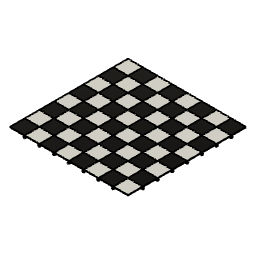
Skak v6 (Autodesk Fusion 360 design; units mm, degrees)
Autodesk Fusion 360 part; units mm, degrees
sketch "Sketch1" plane through (0, 0, 0) normal (1, 0, 0) x (0, 1, 0) in component "Stifner_X"
  line L0 (2, 4) -> (-2, 4)
  line L1 (-2, 4) -> (-2, 0)
  line L2 (-2, 0) -> (2, 0)
  line L3 (2, 0) -> (2, 4)
  dimension "d190" = 4
  dimension "d191" = 4
  constraint horizontal L0
  constraint vertical L1
  constraint horizontal L2
  constraint vertical L3
  constraint midpoint origin L2
  measures "d190" distance of L0 L2
  measures "d191" distance of L0.start L0.end
extrude "Extrude1" add sketch "Sketch1" along normal blind 324 makes body 1 in component "Stifner_X"
sketch "Sketch5" plane through (0, -2, 0) normal (0, -1, 0) x (1, 0, 0) in component "Stifner_X"
  line L0 (0, 4) -> (0, 0)
  line L1 (0, 0) -> (324, 0)
  line L2 (324, 0) -> (324, 4)
  line L3 (324, 4) -> (0, 4)
  line L4 (40, 4) -> (44, 4)
  line L5 (44, 4) -> (44, 2)
  line L6 (44, 2) -> (40, 2)
  line L7 (40, 2) -> (40, 4)
  line L8 (44, 4) -> (44, 2)
  line L9 (44, 2) -> (40, 2)
  line L10 (40, 2) -> (40, 4)
  line L11 (40, 4) -> (44, 4)
  line L12 (80, 2) -> (80, 4)
  line L13 (84, 2) -> (80, 2)
  line L14 (84, 4) -> (84, 2)
  line L15 (80, 4) -> (84, 4)
  line L16 (120, 2) -> (120, 4)
  line L17 (124, 2) -> (120, 2)
  line L18 (124, 4) -> (124, 2)
  line L19 (120, 4) -> (124, 4)
  line L20 (160, 2) -> (160, 4)
  line L21 (164, 2) -> (160, 2)
  line L22 (164, 4) -> (164, 2)
  line L23 (160, 4) -> (164, 4)
  line L24 (200, 2) -> (200, 4)
  line L25 (204, 2) -> (200, 2)
  line L26 (204, 4) -> (204, 2)
  line L27 (200, 4) -> (204, 4)
  line L28 (240, 2) -> (240, 4)
  line L29 (244, 2) -> (240, 2)
  line L30 (244, 4) -> (244, 2)
  line L31 (240, 4) -> (244, 4)
  line L32 (280, 2) -> (280, 4)
  line L33 (284, 2) -> (280, 2)
  line L34 (284, 4) -> (284, 2)
  line L35 (280, 4) -> (284, 4)
  dimension "d200" = 4
  dimension "d201" = 2
  dimension "d202" = 40
  dimension "d205" = 40
  dimension "d206" = 0
  constraint horizontal L4
  constraint vertical L5
  constraint horizontal L6
  constraint vertical L7
  constraint coincident L3 L4.start
  measures "d200" distance of L4.start L4.end
  measures "d201" distance of L4.start L6.end
  measures "d202" distance of L0 L7
extrude "Extrude2" cut sketch "Sketch5" against normal through all contours L3 L4 L5 L6 L7 L8 L9 L10 L11 | L3 L12 L13 L14 L15 | L3 L32 L33 L34 L35 | L3 L16 L17 L18 L19 | L3 L28 L29 L30 L31 | L3 L20 L21 L22 L23 | L3 L24 L25 L26 L27 bodies 1 in component "Stifner_X"
sketch "Sketch1 (2)" plane through (0, 0, 0) normal (0, 1, 0) x (1, 0, 0) in component "Stifner_Y"
  line L0 (-2, -4) -> (2, -4)
  line L1 (2, -4) -> (2, 0)
  line L2 (2, 0) -> (-2, 0)
  line L3 (-2, 0) -> (-2, -4)
  dimension "d207" = 4
  dimension "d208" = 4
  constraint horizontal L0
  constraint vertical L1
  constraint horizontal L2
  constraint vertical L3
  constraint midpoint origin L2
  measures "d207" distance of L0.start L0.end
  measures "d208" distance of L0.start L2.end
extrude "Extrude1'" add sketch "Sketch1 (2)" along normal blind 324 separate body makes body 2 in component "Stifner_Y"
sketch "Sketch3" plane through (2, 0, 0) normal (1, 0, 0) x (0, 1, 0) in component "Stifner_Y"
  line L0 (0, 4) -> (0, 0)
  line L1 (0, 0) -> (324, 0)
  line L2 (324, 0) -> (324, 4)
  line L3 (324, 4) -> (0, 4)
  line L4 (40, 0) -> (44, 0)
  line L5 (44, 0) -> (44, 2)
  line L6 (44, 2) -> (40, 2)
  line L7 (40, 2) -> (40, 0)
  line L8 (40, 0) -> (44, 0)
  line L9 (44, 0) -> (44, 2)
  line L10 (44, 2) -> (40, 2)
  line L11 (40, 2) -> (40, 0)
  line L12 (84, 2) -> (80, 2)
  line L13 (80, 2) -> (80, 0)
  line L14 (80, 0) -> (84, 0)
  line L15 (84, 0) -> (84, 2)
  line L16 (124, 2) -> (120, 2)
  line L17 (120, 2) -> (120, 0)
  line L18 (120, 0) -> (124, 0)
  line L19 (124, 0) -> (124, 2)
  line L20 (164, 2) -> (160, 2)
  line L21 (160, 2) -> (160, 0)
  line L22 (160, 0) -> (164, 0)
  line L23 (164, 0) -> (164, 2)
  line L24 (204, 2) -> (200, 2)
  line L25 (200, 2) -> (200, 0)
  line L26 (200, 0) -> (204, 0)
  line L27 (204, 0) -> (204, 2)
  line L28 (244, 2) -> (240, 2)
  line L29 (240, 2) -> (240, 0)
  line L30 (240, 0) -> (244, 0)
  line L31 (244, 0) -> (244, 2)
  line L32 (284, 2) -> (280, 2)
  line L33 (280, 2) -> (280, 0)
  line L34 (280, 0) -> (284, 0)
  line L35 (284, 0) -> (284, 2)
  point P0 (84, 2)
  point P1 (80, 2)
  point P2 (124, 2)
  point P3 (120, 2)
  point P4 (164, 2)
  point P5 (160, 2)
  point P6 (204, 2)
  point P7 (200, 2)
  point P8 (244, 2)
  point P9 (240, 2)
  point P10 (284, 2)
  point P11 (280, 2)
  dimension "d209" = 2
  dimension "d210" = 4
  dimension "d211" = 40
  dimension "d214" = 40
  dimension "d215" = 0
  dimension "d233" = 0
  constraint horizontal L4
  constraint vertical L5
  constraint horizontal L6
  constraint vertical L7
  constraint coincident L1 L4.start
  measures "d209" distance of L4.start L6.end
  measures "d210" distance of L4.start L4.end
  measures "d211" distance of L0 L7
  measures "d233" distance of L4
extrude "Extrude2'" cut sketch "Sketch3" against normal through all contours L1 L4 L5 L6 L7 L8 L9 L10 L11 | L1 L32 L33 L34 L35 | L1 L12 L13 L14 L15 | L1 L28 L29 L30 L31 | L1 L16 L17 L18 L19 | L1 L24 L25 L26 L27 | L1 L20 L21 L22 L23 bodies 2 in component "Stifner_Y"
pattern_linear "00000000-0000-0000-0000-000000000000" [suppressed]
pattern_linear "00000000-0000-0000-0000-000000000000'" [suppressed]
sketch "Sketch1 (3)" plane through (0, 0, 0) normal (-1, 0, 0) x (0, -1, 0) in component "Edge_X"
  line L0 (-282, 4) -> (42, 4)
  line L1 (42, 4) -> (42, -16)
  line L2 (42, -16) -> (-282, -16)
  line L3 (-282, -16) -> (-282, 4)
  line L4 (42, -2.6667) -> (38, -2.6667)
  line L5 (38, -2.6667) -> (38, -9.3333)
  line L6 (38, -9.3333) -> (42, -9.3333)
  line L7 (42, -9.3333) -> (42, -2.6667)
  line L8 (38, -2.6667) -> (38, 4)
  line L9 (38, -9.3333) -> (38, -16)
  line L10 (-282, -9.3333) -> (-278, -9.3333)
  line L11 (-278, -9.3333) -> (-278, -2.6667)
  line L12 (-278, -2.6667) -> (-282, -2.6667)
  line L13 (-282, -2.6667) -> (-282, -9.3333)
  line L14 (-278, -2.6667) -> (-278, 4)
  line L15 (-278, -9.3333) -> (-278, -16)
  line L16 (-79, 4) -> (-81, 4)
  line L17 (-39, 4) -> (-41, 4)
  line L18 (1, 4) -> (-1, 4)
  line L19 (-119, 4) -> (-121, 4)
  line L20 (-159, 4) -> (-161, 4)
  line L21 (-199, 4) -> (-201, 4)
  line L22 (-239, 4) -> (-241, 4)
  line L23 (-81, 0) -> (-79, 0)
  line L24 (-41, 0) -> (-39, 0)
  line L25 (-1, 0) -> (1, 0)
  line L26 (-121, 0) -> (-119, 0)
  line L27 (-161, 0) -> (-159, 0)
  line L28 (-201, 0) -> (-199, 0)
  line L29 (-241, 0) -> (-239, 0)
  line L30 (-2, 4) -> (-2, 0)
  line L31 (-2, 0) -> (2, 0)
  line L32 (2, 0) -> (2, 4)
  line L33 (2, 4) -> (-2, 4)
  line L34 (-122, 4) -> (-122, 0)
  line L35 (-122, 0) -> (-118, 0)
  line L36 (-118, 0) -> (-118, 4)
  line L37 (-118, 4) -> (-122, 4)
  line L38 (-82, 4) -> (-82, 0)
  line L39 (-82, 0) -> (-78, 0)
  line L40 (-78, 0) -> (-78, 4)
  line L41 (-78, 4) -> (-82, 4)
  line L42 (-42, 4) -> (-42, 0)
  line L43 (-42, 0) -> (-38, 0)
  line L44 (-38, 0) -> (-38, 4)
  line L45 (-38, 4) -> (-42, 4)
  line L46 (-162, 4) -> (-162, 0)
  line L47 (-162, 0) -> (-158, 0)
  line L48 (-158, 0) -> (-158, 4)
  line L49 (-158, 4) -> (-162, 4)
  line L50 (-202, 4) -> (-202, 0)
  line L51 (-202, 0) -> (-198, 0)
  line L52 (-198, 0) -> (-198, 4)
  line L53 (-198, 4) -> (-202, 4)
  line L54 (-242, 4) -> (-242, 0)
  line L55 (-242, 0) -> (-238, 0)
  line L56 (-238, 0) -> (-238, 4)
  line L57 (-238, 4) -> (-242, 4)
  point P0 (-282, -0.2)
  point P1 (42, -0.2)
  dimension "d85" = 20
  dimension "d219" = 4
  dimension "d222" = 4
  constraint horizontal L0
  constraint vertical L1
  constraint horizontal L2
  constraint vertical L3
  constraint horizontal L4
  constraint vertical L5
  constraint horizontal L6
  constraint vertical L7
  constraint coincident L1 L4.start
  constraint coincident L0 L8.end
  constraint perpendicular L0 L8
  constraint coincident L2 L9.end
  constraint perpendicular L2 L9
  constraint equal L5 L9
  constraint equal L5 L8
  constraint horizontal L10
  constraint vertical L11
  constraint horizontal L12
  constraint vertical L13
  constraint coincident L3 L10.start
  constraint coincident L0 L14.end
  constraint perpendicular L0 L14
  constraint coincident L2 L15.end
  constraint perpendicular L2 L15
  constraint equal L11 L15
  constraint equal L11 L14
  constraint coincident L0 L22.start
  constraint coincident L3 P0
  constraint coincident L1 P1
  measures "d85" distance of L2.end L0.start
  measures "d219" distance of L11.end L12.end
  measures "d222" distance of L4.start L4.end
extrude "Extrude2''" add sketch "Sketch1 (3)" against normal blind 4 separate body contours L0 L2 L5 L8 L9 L11 L14 L15 L23 L24 L25 L26 L27 L28 L29 L30 L31 L32 L34 L35 L36 L38 L39 L40 L42 L43 L44 L46 L47 L48 L50 L51 L52 L54 L55 L56 | L3 L10 L11 L12 L13 | L1 L2 L6 L9 | L0 L1 L4 L8 makes body 3 in component "Edge_X"
sketch "Sketch1 (4)" plane through (-2, 282, -0.2) normal (0, -1, 0) x (1, 0, 0) in component "Edge_Y"
  line L0 (6, 4) -> (322, 4)
  line L1 (322, 4) -> (322, -16)
  line L2 (322, -16) -> (6, -16)
  line L3 (6, -16) -> (6, 4)
  line L4 (45, 4) -> (43, 4)
  line L5 (85, 4) -> (83, 4)
  line L6 (125, 4) -> (123, 4)
  line L7 (165, 4) -> (163, 4)
  line L8 (205, 4) -> (203, 4)
  line L9 (245, 4) -> (243, 4)
  line L10 (285, 4) -> (283, 4)
  line L11 (43, 0) -> (45, 0)
  line L12 (83, 0) -> (85, 0)
  line L13 (123, 0) -> (125, 0)
  line L14 (163, 0) -> (165, 0)
  line L15 (203, 0) -> (205, 0)
  line L16 (243, 0) -> (245, 0)
  line L17 (283, 0) -> (285, 0)
  line L18 (122, 0) -> (122, 4)
  line L19 (122, 4) -> (126, 4)
  line L20 (126, 4) -> (126, 0)
  line L21 (126, 0) -> (122, 0)
  line L22 (2, -2.4667) -> (2, 4.2)
  line L23 (2, 4.2) -> (6, 4.2)
  line L24 (6, 4.2) -> (6, -2.4667)
  line L25 (6, -2.4667) -> (2, -2.4667)
  line L26 (2, -15.8) -> (2, -9.1333)
  line L27 (2, -9.1333) -> (6, -9.1333)
  line L28 (6, -9.1333) -> (6, -15.8)
  line L29 (6, -15.8) -> (2, -15.8)
  line L30 (326, -2.4667) -> (326, -9.1333)
  line L31 (326, -9.1333) -> (322, -9.1333)
  line L32 (322, -9.1333) -> (322, -2.4667)
  line L33 (322, -2.4667) -> (326, -2.4667)
  line L34 (282, 0) -> (282, 4)
  line L35 (282, 4) -> (286, 4)
  line L36 (286, 4) -> (286, 0)
  line L37 (286, 0) -> (282, 0)
  line L38 (242, 0) -> (242, 4)
  line L39 (242, 4) -> (246, 4)
  line L40 (246, 4) -> (246, 0)
  line L41 (246, 0) -> (242, 0)
  line L42 (202, 0) -> (202, 4)
  line L43 (202, 4) -> (206, 4)
  line L44 (206, 4) -> (206, 0)
  line L45 (206, 0) -> (202, 0)
  line L46 (162, 0) -> (162, 4)
  line L47 (162, 4) -> (166, 4)
  line L48 (166, 4) -> (166, 0)
  line L49 (166, 0) -> (162, 0)
  line L50 (122, 2) -> (122, 0)
  line L51 (122, 0) -> (126, 0)
  line L52 (126, 0) -> (126, 2)
  line L53 (126, 2) -> (122, 2)
  line L54 (82, 0) -> (82, 4)
  line L55 (82, 4) -> (86, 4)
  line L56 (86, 4) -> (86, 0)
  line L57 (86, 0) -> (82, 0)
  line L58 (122, 4) -> (122, 0)
  line L59 (122, 0) -> (126, 0)
  line L60 (126, 0) -> (126, 4)
  line L61 (126, 4) -> (122, 4)
  line L62 (42, 0) -> (42, 4)
  line L63 (42, 4) -> (46, 4)
  line L64 (46, 4) -> (46, 0)
  line L65 (46, 0) -> (42, 0)
  constraint horizontal L0
  constraint vertical L1
  constraint horizontal L2
  constraint vertical L3
  constraint coincident L0 L4.end
  constraint coincident L1 L32.end
  constraint coincident L3 L24.end
extrude "Extrude1''" add sketch "Sketch1 (4)" along normal blind 4 separate body contours L0 L1 L2 L3 L11 L12 L13 L14 L15 L16 L17 L18 L20 L21 L24 L28 L32 L34 L36 L37 L38 L40 L41 L42 L44 L45 L46 L48 L49 L50 L51 L52 L54 L56 L57 L58 L59 L60 L62 L64 L65 | L3 L22 L23 L24 L25 | L3 L26 L27 L28 L29 | L1 L30 L31 L32 L33 makes body 4 in component "Edge_Y"
sketch "Sketch3 (2)" plane through (0, -45, 3.8) normal (0, 0, 1) x (-1, 0, 0) in component "Tile"
  line L0 (-4, -323) -> (-40, -323)
  line L1 (-2, -45) -> (-42, -45)
  line L2 (-42, -45) -> (-42, -5)
  line L3 (-42, -5) -> (-2, -5)
  line L4 (-2, -5) -> (-2, -45)
  line L5 (-320, -323) -> (-320, -327)
  line L6 (-124, -327) -> (-124, -323)
  line L7 (-84, -323) -> (-120, -323)
  line L8 (-120, -323) -> (-120, -327)
  line L9 (-40, -3) -> (-40, -327)
  line L10 (0, -43) -> (-40, -43)
  line L11 (-204, -327) -> (-204, -323)
  line L12 (-240, -323) -> (-240, -327)
  line L13 (-40, -327) -> (-4, -327)
  line L14 (-44, -327) -> (-44, -323)
  line L15 (-44, -323) -> (-80, -323)
  line L16 (-80, -323) -> (-80, -327)
  line L17 (-120, -327) -> (-84, -327)
  line L18 (-84, -327) -> (-84, -323)
  line L19 (-160, -327) -> (-124, -327)
  line L20 (-124, -323) -> (-160, -323)
  line L21 (-160, -323) -> (-160, -327)
  line L22 (-200, -327) -> (-164, -327)
  line L23 (-164, -327) -> (-164, -323)
  line L24 (-164, -323) -> (-200, -323)
  line L25 (-200, -323) -> (-200, -327)
  line L26 (-280, -327) -> (-244, -327)
  line L27 (-244, -327) -> (-244, -323)
  line L28 (-244, -323) -> (-280, -323)
  line L29 (-280, -323) -> (-280, -327)
  line L30 (-320, -327) -> (-284, -327)
  line L31 (-284, -327) -> (-284, -323)
  line L32 (-284, -323) -> (-320, -323)
  line L33 (-44, -327) -> (-80, -327)
  line L34 (-124, -327) -> (-160, -327)
  line L35 (-244, -327) -> (-280, -327)
  line L36 (-284, -327) -> (-320, -327)
  line L37 (-84, -327) -> (-120, -327)
  line L38 (-204, -327) -> (-240, -327)
  line L39 (-164, -327) -> (-200, -327)
  line L40 (-240, -327) -> (-204, -327)
  line L41 (-4, -327) -> (-4, -323)
  line L42 (-40, -323) -> (-40, -327)
  line L43 (-204, -323) -> (-240, -323)
  line L44 (-80, -327) -> (-44, -327)
  line L45 (-4, -327) -> (-40, -327)
  dimension "d161" = 40
  dimension "d162" = 40
  dimension "d223" = 2
  dimension "d224" = 2
  constraint horizontal L1
  constraint vertical L2
  constraint horizontal L3
  constraint vertical L4
  measures "d161" distance of L1.start L1.end
  measures "d162" distance of L1.start L3.end
  measures "d223" distance of L2 L9
  measures "d224" distance of L1 L10
extrude "Extrude2'''" add sketch "Sketch3 (2)" along normal blind 2 separate body contours L1 L4 L9 L10 | L1 L2 L3 L9 | L3 L4 L9 L10 makes body 5 in component "Tile"
pattern_linear "00000000-0000-0000-0000-000000000000''" [suppressed] in component "Tiles"
sketch "Sketch7" plane through (0, 0, 3.8) normal (0, 0, -1) x (1, 0, 0) in component "Tile"
  line L0 (42, 40) -> (2, 40)
  line L1 (2, 40) -> (2, 0)
  line L2 (2, 0) -> (42, 0)
  line L3 (42, 0) -> (42, 40)
  line L4 (4, 2) -> (40, 2)
  line L5 (40, 2) -> (40, 38)
  line L6 (40, 38) -> (4, 38)
  line L7 (4, 38) -> (4, 2)
  dimension "d243" = -2
extrude "Extrude5" add sketch "Sketch7" along normal blind 2 contours L4 L5 L6 L7 bodies 5 in component "Tile"
sketch "Sketch6" plane through (0, 0, 5.8) normal (0, 0, 1) x (-1, 0, 0) in component "Tile"
  line L0 (-2, 40) -> (-42, 40)
  line L1 (-42, 40) -> (-42, 0)
  line L2 (-42, 0) -> (-2, 0)
  line L3 (-2, 0) -> (-2, 40)
  line L4 (-22, 0) -> (-22, 40) construction
  line L5 (-42, 20) -> (-2, 20) construction
  line L6 (-16, 19.25) -> (-28, 19.25)
  line L7 (-28, 19.25) -> (-28, 20.75)
  line L8 (-28, 20.75) -> (-16, 20.75)
  line L9 (-16, 20.75) -> (-16, 19.25)
  line L10 (-16, 19.25) -> (-28, 20.75) construction
  line L11 (-21.25, 14) -> (-22.75, 14)
  line L12 (-22.75, 14) -> (-22.75, 18)
  line L13 (-22.75, 18) -> (-21.25, 18)
  line L14 (-21.25, 18) -> (-21.25, 14)
  line L15 (-22.75, 22) -> (-21.25, 22)
  line L16 (-22.75, 26) -> (-22.75, 22)
  line L17 (-21.25, 26) -> (-22.75, 26)
  line L18 (-21.25, 22) -> (-21.25, 26)
  point P0 (-22, 20)
  dimension "d183" = 12
  dimension "d184" = 1.5
  dimension "d185" = 1.5
  dimension "d186" = 4
  dimension "d187" = 2
  constraint midpoint L2 L4.start
  constraint midpoint L0 L4.end
  constraint midpoint L1 L5.start
  constraint midpoint L3 L5.end
  constraint horizontal L6
  constraint vertical L7
  constraint horizontal L8
  constraint vertical L9
  constraint midpoint L4 P0
  constraint midpoint L10 P0
  constraint horizontal L11
  constraint vertical L12
  constraint horizontal L13
  constraint vertical L14
  constraint symmetric L4 L12 L14
  constraint symmetric L5 L11.start L17.start
  constraint symmetric L5 L11.end L16.start
  constraint symmetric L5 L12.end L15.start
  constraint symmetric L5 L13.end L15.end
  measures "d183" distance of L6.start L6.end
  measures "d184" distance of L6.start L8.end
  measures "d185" distance of L11.start L11.end
  measures "d186" distance of L11.start L13.end
  measures "d187" distance of L5 L13
extrude "Extrude4" add sketch "Sketch6" along normal blind 0.5 separate body contours L6 L7 L8 L9 | L11 L12 L13 L14 | L15 L16 L17 L18 makes body 6 at (24, -20.25, 5.8) makes body 7 at (21.75, -15.3333, 5.8) makes body 8 at (22.25, -24.6667, 5.8) in component "Tile"
component "Edges" placed x (1, 0, 0) y (0, 1, 0) z (0, 0, 1) at (0, 0, 0)
component "Stifner_X_all" placed x (1, 0, 0) y (0, 1, 0) z (0, 0, 1) at (0, 0, 0)
component "Stifner_Y_all" placed x (1, 0, 0) y (0, 1, 0) z (0, 0, 1) at (0, 0, 0)
component "Tiles" placed x (1, 0, 0) y (0, 1, 0) z (0, 0, 1) at (0, 0, 0)
component "Edge_X" placed x (1, 0, 0) y (0, 1, 0) z (0, 0, 1) at (0, 0, 0) in component "Edges"
component "Edge_X" placed x (-1, 0, 0) y (0, -1, 0) z (0, 0, 1) at (324, 240, 0) in component "Edges"
component "Edge_Y" placed x (1, 0, 0) y (0, 1, 0) z (0, 0, 1) at (0, 0, 0) in component "Edges"
component "Edge_Y" placed x (-1, 0, 0) y (0, -1, 0) z (0, 0, 1) at (324, 240, 0) in component "Edges"
component "Stifner_X" placed x (1, 0, 0) y (0, 1, 0) z (0, 0, 1) at (0, 240, 0) in component "Stifner_X_all"
component "Stifner_X" placed x (1, 0, 0) y (0, 1, 0) z (0, 0, 1) at (0, 200, 0) in component "Stifner_X_all"
component "Stifner_X" placed x (1, 0, 0) y (0, 1, 0) z (0, 0, 1) at (0, 160, 0) in component "Stifner_X_all"
component "Stifner_X" placed x (1, 0, 0) y (0, 1, 0) z (0, 0, 1) at (0, 120, 0) in component "Stifner_X_all"
component "Stifner_X" placed x (1, 0, 0) y (0, 1, 0) z (0, 0, 1) at (0, 0, 0) in component "Stifner_X_all"
component "Stifner_X" placed x (1, 0, 0) y (0, 1, 0) z (0, 0, 1) at (0, 40, 0) in component "Stifner_X_all"
component "Stifner_X" placed x (1, 0, 0) y (0, 1, 0) z (0, 0, 1) at (0, 80, 0) in component "Stifner_X_all"
component "Stifner_Y" placed x (1, 0, 0) y (0, 1, 0) z (0, 0, 1) at (282, -42, -0.2) in component "Stifner_Y_all"
component "Stifner_Y" placed x (1, 0, 0) y (0, 1, 0) z (0, 0, 1) at (42, -42, -0.2) in component "Stifner_Y_all"
component "Stifner_Y" placed x (1, 0, 0) y (0, 1, 0) z (0, 0, 1) at (82, -42, -0.2) in component "Stifner_Y_all"
component "Stifner_Y" placed x (1, 0, 0) y (0, 1, 0) z (0, 0, 1) at (122, -42, -0.2) in component "Stifner_Y_all"
component "Stifner_Y" placed x (1, 0, 0) y (0, 1, 0) z (0, 0, 1) at (162, -42, -0.2) in component "Stifner_Y_all"
component "Stifner_Y" placed x (1, 0, 0) y (0, 1, 0) z (0, 0, 1) at (202, -42, -0.2) in component "Stifner_Y_all"
component "Stifner_Y" placed x (1, 0, 0) y (0, 1, 0) z (0, 0, 1) at (242, -42, -0.2) in component "Stifner_Y_all"
component "Tile" placed x (1, 0, 0) y (0, 1, 0) z (0, 0, 1) at (0, 0, 0.2) in component "Tiles"
component "Tile" placed x (1, 0, 0) y (0, 1, 0) z (0, 0, 1) at (40, 0, 0.2) in component "Tiles"
component "Tile" placed x (1, 0, 0) y (0, 1, 0) z (0, 0, 1) at (80, 0, 0.2) in component "Tiles"
component "Tile" placed x (1, 0, 0) y (0, 1, 0) z (0, 0, 1) at (120, 0, 0.2) in component "Tiles"
component "Tile" placed x (1, 0, 0) y (0, 1, 0) z (0, 0, 1) at (160, 0, 0.2) in component "Tiles"
component "Tile" placed x (1, 0, 0) y (0, 1, 0) z (0, 0, 1) at (200, 0, 0.2) in component "Tiles"
component "Tile" placed x (1, 0, 0) y (0, 1, 0) z (0, 0, 1) at (240, 0, 0.2) in component "Tiles"
component "Tile" placed x (1, 0, 0) y (0, 1, 0) z (0, 0, 1) at (280, 0, 0.2) in component "Tiles"
component "Tile" placed x (1, 0, 0) y (0, 1, 0) z (0, 0, 1) at (0, 40, 0.2) in component "Tiles"
component "Tile" placed x (1, 0, 0) y (0, 1, 0) z (0, 0, 1) at (40, 40, 0.2) in component "Tiles"
component "Tile" placed x (1, 0, 0) y (0, 1, 0) z (0, 0, 1) at (80, 40, 0.2) in component "Tiles"
component "Tile" placed x (1, 0, 0) y (0, 1, 0) z (0, 0, 1) at (120, 40, 0.2) in component "Tiles"
component "Tile" placed x (1, 0, 0) y (0, 1, 0) z (0, 0, 1) at (160, 40, 0.2) in component "Tiles"
component "Tile" placed x (1, 0, 0) y (0, 1, 0) z (0, 0, 1) at (200, 40, 0.2) in component "Tiles"
component "Tile" placed x (1, 0, 0) y (0, 1, 0) z (0, 0, 1) at (240, 40, 0.2) in component "Tiles"
component "Tile" placed x (1, 0, 0) y (0, 1, 0) z (0, 0, 1) at (280, 40, 0.2) in component "Tiles"
component "Tile" placed x (1, 0, 0) y (0, 1, 0) z (0, 0, 1) at (0, 80, 0.2) in component "Tiles"
component "Tile" placed x (1, 0, 0) y (0, 1, 0) z (0, 0, 1) at (40, 80, 0.2) in component "Tiles"
component "Tile" placed x (1, 0, 0) y (0, 1, 0) z (0, 0, 1) at (80, 80, 0.2) in component "Tiles"
component "Tile" placed x (1, 0, 0) y (0, 1, 0) z (0, 0, 1) at (120, 80, 0.2) in component "Tiles"
component "Tile" placed x (1, 0, 0) y (0, 1, 0) z (0, 0, 1) at (160, 80, 0.2) in component "Tiles"
component "Tile" placed x (1, 0, 0) y (0, 1, 0) z (0, 0, 1) at (200, 80, 0.2) in component "Tiles"
component "Tile" placed x (1, 0, 0) y (0, 1, 0) z (0, 0, 1) at (240, 80, 0.2) in component "Tiles"
component "Tile" placed x (1, 0, 0) y (0, 1, 0) z (0, 0, 1) at (280, 80, 0.2) in component "Tiles"
component "Tile" placed x (1, 0, 0) y (0, 1, 0) z (0, 0, 1) at (0, 120, 0.2) in component "Tiles"
component "Tile" placed x (1, 0, 0) y (0, 1, 0) z (0, 0, 1) at (40, 120, 0.2) in component "Tiles"
component "Tile" placed x (1, 0, 0) y (0, 1, 0) z (0, 0, 1) at (80, 120, 0.2) in component "Tiles"
component "Tile" placed x (1, 0, 0) y (0, 1, 0) z (0, 0, 1) at (120, 120, 0.2) in component "Tiles"
component "Tile" placed x (1, 0, 0) y (0, 1, 0) z (0, 0, 1) at (160, 120, 0.2) in component "Tiles"
component "Tile" placed x (1, 0, 0) y (0, 1, 0) z (0, 0, 1) at (200, 120, 0.2) in component "Tiles"
component "Tile" placed x (1, 0, 0) y (0, 1, 0) z (0, 0, 1) at (240, 120, 0.2) in component "Tiles"
component "Tile" placed x (1, 0, 0) y (0, 1, 0) z (0, 0, 1) at (280, 120, 0.2) in component "Tiles"
component "Tile" placed x (1, 0, 0) y (0, 1, 0) z (0, 0, 1) at (0, 160, 0.2) in component "Tiles"
component "Tile" placed x (1, 0, 0) y (0, 1, 0) z (0, 0, 1) at (40, 160, 0.2) in component "Tiles"
component "Tile" placed x (1, 0, 0) y (0, 1, 0) z (0, 0, 1) at (80, 160, 0.2) in component "Tiles"
component "Tile" placed x (1, 0, 0) y (0, 1, 0) z (0, 0, 1) at (120, 160, 0.2) in component "Tiles"
component "Tile" placed x (1, 0, 0) y (0, 1, 0) z (0, 0, 1) at (160, 160, 0.2) in component "Tiles"
component "Tile" placed x (1, 0, 0) y (0, 1, 0) z (0, 0, 1) at (200, 160, 0.2) in component "Tiles"
component "Tile" placed x (1, 0, 0) y (0, 1, 0) z (0, 0, 1) at (240, 160, 0.2) in component "Tiles"
component "Tile" placed x (1, 0, 0) y (0, 1, 0) z (0, 0, 1) at (280, 160, 0.2) in component "Tiles"
component "Tile" placed x (1, 0, 0) y (0, 1, 0) z (0, 0, 1) at (0, 200, 0.2) in component "Tiles"
component "Tile" placed x (1, 0, 0) y (0, 1, 0) z (0, 0, 1) at (40, 200, 0.2) in component "Tiles"
component "Tile" placed x (1, 0, 0) y (0, 1, 0) z (0, 0, 1) at (80, 200, 0.2) in component "Tiles"
component "Tile" placed x (1, 0, 0) y (0, 1, 0) z (0, 0, 1) at (120, 200, 0.2) in component "Tiles"
component "Tile" placed x (1, 0, 0) y (0, 1, 0) z (0, 0, 1) at (160, 200, 0.2) in component "Tiles"
component "Tile" placed x (1, 0, 0) y (0, 1, 0) z (0, 0, 1) at (200, 200, 0.2) in component "Tiles"
component "Tile" placed x (1, 0, 0) y (0, 1, 0) z (0, 0, 1) at (240, 200, 0.2) in component "Tiles"
component "Tile" placed x (1, 0, 0) y (0, 1, 0) z (0, 0, 1) at (280, 200, 0.2) in component "Tiles"
component "Tile" placed x (1, 0, 0) y (0, 1, 0) z (0, 0, 1) at (0, 240, 0.2) in component "Tiles"
component "Tile" placed x (1, 0, 0) y (0, 1, 0) z (0, 0, 1) at (40, 240, 0.2) in component "Tiles"
component "Tile" placed x (1, 0, 0) y (0, 1, 0) z (0, 0, 1) at (80, 240, 0.2) in component "Tiles"
component "Tile" placed x (1, 0, 0) y (0, 1, 0) z (0, 0, 1) at (120, 240, 0.2) in component "Tiles"
component "Tile" placed x (1, 0, 0) y (0, 1, 0) z (0, 0, 1) at (160, 240, 0.2) in component "Tiles"
component "Tile" placed x (1, 0, 0) y (0, 1, 0) z (0, 0, 1) at (200, 240, 0.2) in component "Tiles"
component "Tile" placed x (1, 0, 0) y (0, 1, 0) z (0, 0, 1) at (240, 240, 0.2) in component "Tiles"
component "Tile" placed x (1, 0, 0) y (0, 1, 0) z (0, 0, 1) at (280, 240, 0.2) in component "Tiles"
component "Tile" placed x (1, 0, 0) y (0, 1, 0) z (0, 0, 1) at (0, 280, 0.2) in component "Tiles"
component "Tile" placed x (1, 0, 0) y (0, 1, 0) z (0, 0, 1) at (40, 280, 0.2) in component "Tiles"
component "Tile" placed x (1, 0, 0) y (0, 1, 0) z (0, 0, 1) at (80, 280, 0.2) in component "Tiles"
component "Tile" placed x (1, 0, 0) y (0, 1, 0) z (0, 0, 1) at (120, 280, 0.2) in component "Tiles"
component "Tile" placed x (1, 0, 0) y (0, 1, 0) z (0, 0, 1) at (160, 280, 0.2) in component "Tiles"
component "Tile" placed x (1, 0, 0) y (0, 1, 0) z (0, 0, 1) at (200, 280, 0.2) in component "Tiles"
component "Tile" placed x (1, 0, 0) y (0, 1, 0) z (0, 0, 1) at (240, 280, 0.2) in component "Tiles"
component "Tile" placed x (1, 0, 0) y (0, 1, 0) z (0, 0, 1) at (280, 280, 0.2) in component "Tiles"
hidden bodies 6 7 8
equation "stifner_thickness = 4 mm"
equation "stifner_height = 4 mm"
equation "stifner_fod_with = 8 mm"
equation "tile_with = 40 mm"
equation "d10 = tile_with * 8 + 2 * overhang_edge - stifner_thickness"
equation "d27 = 8 * tile_with + 2 * overhang_edge - stifner_thickness"
equation "overhang_edge = 4 mm"
equation "d70 = 2 * offset"
equation "d73 = tile_with"
equation "d77 = tile_with"
equation "d161 = tile_with - offset * 2"
equation "d162 = tile_with - offset * 2"
equation "d165 = stifner_thickness / 2"
equation "d177 = tile_with"
equation "d178 = tile_with"
equation "d190 = stifner_height"
equation "d191 = stifner_thickness"
equation "d200 = stifner_thickness"
equation "d201 = stifner_height / 2"
equation "d202 = overhang_edge + tile_with - stifner_thickness"
equation "d205 = tile_with"
equation "d207 = stifner_thickness"
equation "d208 = stifner_height"
equation "d209 = stifner_height / 2"
equation "d210 = stifner_thickness"
equation "d211 = overhang_edge + tile_with - stifner_thickness"
equation "d214 = tile_with"
equation "d218 = overhang_edge"
equation "d219 = overhang_edge"
equation "d220 = -overhang_edge"
equation "d222 = overhang_edge"
equation "d223 = stifner_thickness / 2 - offset"
equation "d224 = stifner_thickness / 2 - offset"
equation "d226 = overhang_edge - stifner_thickness / 2"
equation "d227 = overhang_edge - stifner_thickness / 2"
equation "d229 = stifner_height / 2"
equation "offset = 0 mm"
equation "d232 = -offset"
equation "d233 = offset"
equation "d243 = -stifner_thickness / 2"
